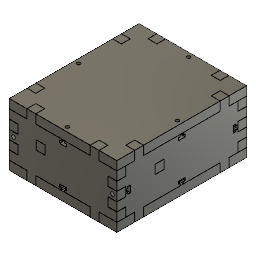
Basic-Case_1_ (Autodesk Fusion 360 design; units mm, degrees)
Autodesk Fusion 360 part; units mm, degrees
sketch "Sketch1" plane through (0, 0, 0) normal (0, 1, 0) x (1, 0, 0)
  line L0 (20, -25) -> (-20, -25) construction
  line L1 (-20, -25) -> (-20, 25) construction
  line L2 (-20, 25) -> (20, 25) construction
  line L3 (20, 25) -> (20, -25) construction
  line L4 (20, -25) -> (-20, 25) construction
  line L5 (-20, -25) -> (20, 25) construction
  line L6 (-20.2, -25.2) -> (-20.2, 25.2)
  line L7 (-20.2, 25.2) -> (20.2, 25.2)
  line L8 (20.2, 25.2) -> (20.2, -25.2)
  line L9 (20.2, -25.2) -> (-20.2, -25.2)
  line L10 (-24.2, -29.2) -> (-24.2, 29.2)
  line L11 (-24.2, 29.2) -> (24.2, 29.2)
  line L12 (24.2, 29.2) -> (24.2, -29.2)
  line L13 (24.2, -29.2) -> (-24.2, -29.2)
  line L14 (-101.376, 37.6811) -> (-97.376, 37.6811)
  circle A0 centre (-145.6614, -116.3344) radius 0.8
  line L15 (-102.0936, 18.9478) -> (-98.0936, 18.9478) construction
  line L16 (-115.2743, 43.6415) -> (-83.6806, 43.6415) construction
  line L17 (-83.6806, 43.6415) -> (-83.6806, 47.6415) construction
  line L18 (-83.6806, 47.6415) -> (-115.2743, 47.6415) construction
  line L19 (-115.2743, 47.6415) -> (-115.2743, 43.6415) construction
  line L20 (-141.8809, -116.5884) -> (-121.0391, -116.5884) construction
  line L21 (-121.0391, -116.5884) -> (-121.0391, -112.5884) construction
  line L22 (-121.0391, -112.5884) -> (-141.8809, -112.5884) construction
  line L23 (-141.8809, -112.5884) -> (-141.8809, -116.5884) construction
  line L24 (-113.6442, 20.144) -> (-90.9391, 20.144) construction
  line L25 (-90.9391, 20.144) -> (-90.9391, 24.144) construction
  line L26 (-90.9391, 24.144) -> (-113.6442, 24.144) construction
  line L27 (-113.6442, 24.144) -> (-113.6442, 20.144) construction
  line L28 (-117.1274, 62.4181) -> (-97.1274, 62.4181) construction
  line L29 (-106.7649, 64.5631) -> (-88.5969, 64.5631) construction
  line L30 (-88.5969, 64.5631) -> (-88.5969, 68.5631) construction
  line L31 (-88.5969, 68.5631) -> (-106.7649, 68.5631) construction
  line L32 (-106.7649, 68.5631) -> (-106.7649, 64.5631) construction
  line L33 (-131.4609, -76.5113) -> (-128.4609, -76.5113) construction
  line L34 (-133.0423, -91.4513) -> (-131.8423, -91.4513) construction
  line L35 (-127.3164, -91.6771) -> (-110.039, -91.6771) construction
  line L36 (-110.039, -91.6771) -> (-110.039, -87.6771) construction
  line L37 (-110.039, -87.6771) -> (-127.3164, -87.6771) construction
  line L38 (-127.3164, -87.6771) -> (-127.3164, -91.6771) construction
  line L39 (-126.3991, -76.4909) -> (-110.9245, -76.4909) construction
  line L40 (-110.9245, -76.4909) -> (-110.9245, -72.4909) construction
  line L41 (-110.9245, -72.4909) -> (-126.3991, -72.4909) construction
  line L42 (-126.3991, -72.4909) -> (-126.3991, -76.4909) construction
  line L43 (-135.3666, -105.8982) -> (-129.2666, -105.8982) construction
  line L44 (-125.3145, -106.1826) -> (-103.254, -106.1826) construction
  line L45 (-103.254, -106.1826) -> (-103.254, -102.1826) construction
  line L46 (-103.254, -102.1826) -> (-125.3145, -102.1826) construction
  line L47 (-125.3145, -102.1826) -> (-125.3145, -106.1826) construction
  dimension "d1" = 50
  dimension "d2" = 40
  dimension "d3" = 0.2
  dimension "d4" = 4.2
  dimension "d9" = 4
  dimension "d141" = 1.6
  dimension "d199" = 4
  dimension "d225" = 20
  dimension "d273" = 6.1
  dimension "d274" = 1.2
  dimension "d275" = 3
  constraint perpendicular L0 L1
  constraint parallel L0 L2
  constraint parallel L1 L3
  constraint horizontal L0
  constraint coincident L4 origin
  constraint coincident L5 origin
  constraint horizontal L14
  constraint horizontal L15
  constraint perpendicular L16 L17
  constraint parallel L16 L18
  constraint parallel L17 L19
  constraint perpendicular L20 L21
  constraint parallel L20 L22
  constraint parallel L21 L23
  constraint perpendicular L24 L25
  constraint parallel L24 L26
  constraint parallel L25 L27
  constraint horizontal L28
  constraint perpendicular L29 L30
  constraint parallel L29 L31
  constraint parallel L30 L32
  constraint horizontal L33
  constraint horizontal L34
  constraint perpendicular L35 L36
  constraint parallel L35 L37
  constraint parallel L36 L38
  constraint perpendicular L39 L40
  constraint parallel L39 L41
  constraint parallel L40 L42
  constraint horizontal L43
  constraint perpendicular L44 L45
  constraint parallel L44 L46
  constraint parallel L45 L47
  measures "d1" distance of L0.start L2.end
  measures "d2" distance of L0.start L0.end
  measures "d9" distance of L14.start L14.end
  measures "d141" diameter of A0
  measures "d199" distance of L15.start L15.end
  measures "d225" distance of L28.start L28.end
  measures "d273" distance of L43.start L43.end
  measures "d274" distance of L34.start L34.end
  measures "d275" distance of L33.start L33.end
extrude "Extrude1" add sketch "Sketch1" against normal blind 4 contours L6 L7 L8 L9 | L10 L11 L12 L13 makes body 1
extrude "Extrude3" add sketch "Sketch1" along normal blind 20 separate body contours L10 L11 L12 L13 makes body 2
sketch "Sketch2" plane through (0, 20, 0) normal (0, 1, 0) x (-1, 0, 0)
  line L0 (-20.2, -25.2) -> (-20.2, 25.2)
  line L1 (-20.2, 25.2) -> (20.2, 25.2)
  line L2 (20.2, 25.2) -> (20.2, -25.2)
  line L3 (20.2, -25.2) -> (-20.2, -25.2)
  line L4 (-24.2, 29.2) -> (-24.2, -29.2)
  line L5 (-24.2, -29.2) -> (24.2, -29.2)
  line L6 (24.2, -29.2) -> (24.2, 29.2)
  line L7 (24.2, 29.2) -> (-24.2, 29.2)
  line L8 (20.2, -25.2) -> (24.2, -29.2) construction
  line L9 (-20.2, -25.2) -> (-24.2, -29.2) construction
  line L10 (-20.2, 25.2) -> (-24.2, 29.2) construction
  line L11 (20.2, 25.2) -> (24.2, 29.2) construction
  circle A0 centre (22.2, 27.2) radius 0.75
  circle A1 centre (-22.2, 27.2) radius 0.75
  circle A2 centre (-22.2, -27.2) radius 0.75
  circle A3 centre (22.2, -27.2) radius 0.75
  dimension "d95" = 1.5
  dimension "d96" = 1.5
  dimension "d97" = 1.5
  dimension "d98" = 1.5
  constraint coincident L2.end L3.start
  constraint coincident L5.end L6.start
  constraint coincident L0.start L3.end
  constraint coincident L4.end L5.start
  constraint coincident L0.end L1.start
  constraint coincident L4.start L7.end
  constraint coincident L1.end L2.start
  constraint coincident L6.end L7.start
  constraint midpoint L11 A0.centre
  constraint midpoint L10 A1.centre
  constraint midpoint L9 A2.centre
  constraint midpoint L8 A3.centre
  measures "d95" diameter of A0
  measures "d96" diameter of A1
  measures "d97" diameter of A2
  measures "d98" diameter of A3
extrude "Extrude4" add sketch "Sketch2" along normal blind 4 separate body contours L0 L1 L2 L3 | L4 L5 L6 L7 | A0 | A1 | A2 | A3 makes body 3
sketch "Sketch7" plane through (0, 20, 0) normal (0, 1, 0) x (-1, 0, 0)
  line L0 (24.2, -29.2) -> (24.2, 29.2)
  line L1 (24.2, 29.2) -> (-24.2, 29.2)
  line L2 (-24.2, 29.2) -> (-24.2, -29.2)
  line L3 (-24.2, -29.2) -> (24.2, -29.2)
  line L4 (-20.2, -25.2) -> (-20.2, 25.2)
  line L5 (-20.2, 25.2) -> (20.2, 25.2)
  line L6 (20.2, 25.2) -> (20.2, -25.2)
  line L7 (20.2, -25.2) -> (-20.2, -25.2)
  line L8 (-12.2, -25.2) -> (-16.2, -25.2)
  line L9 (-16.2, -25.2) -> (-16.2, -29.2)
  line L10 (-16.2, -29.2) -> (-12.2, -29.2)
  line L11 (-12.2, -29.2) -> (-12.2, -25.2)
  line L12 (-24.2, -17.2) -> (-20.2, -17.2)
  line L13 (-20.2, -17.2) -> (-20.2, -21.2)
  line L14 (-20.2, -21.2) -> (-24.2, -21.2)
  line L15 (-24.2, -21.2) -> (-24.2, -17.2)
  line L16 (-24.2, 21.2) -> (-20.2, 21.2)
  line L17 (-24.2, 17.2) -> (-20.2, 17.2)
  line L18 (-16.2, 25.2) -> (-16.2, 29.2)
  line L19 (-12.2, 29.2) -> (-12.2, 25.2)
  line L20 (16.2, 29.2) -> (16.2, 25.2)
  line L21 (12.2, 25.2) -> (12.2, 29.2)
  line L22 (20.2, 21.2) -> (24.2, 21.2)
  line L23 (24.2, 17.2) -> (20.2, 17.2)
  line L24 (12.2, -25.2) -> (12.2, -29.2)
  line L25 (16.2, -25.2) -> (16.2, -29.2)
  line L26 (20.2, -21.2) -> (24.2, -21.2)
  line L27 (24.2, -17.2) -> (20.2, -17.2)
  line L28 (24.2, 0) -> (-24.2, 0) construction
  dimension "d74" = 4
  dimension "d75" = 4
  dimension "d76" = 4
  dimension "d77" = 4
  dimension "d78" = 4
  dimension "d79" = 4
  dimension "d80" = 4
  dimension "d81" = 4
  dimension "d82" = 4
  dimension "d83" = 4
  dimension "d84" = 4
  dimension "d85" = 4
  dimension "d86" = 4
  dimension "d87" = 4
  dimension "d88" = 4
  dimension "d198" = 4
  constraint horizontal L8
  constraint vertical L9
  constraint horizontal L10
  constraint vertical L11
  constraint coincident L3 L9.end
  constraint horizontal L12
  constraint vertical L13
  constraint horizontal L14
  constraint vertical L15
  constraint coincident L4 L13.end
  constraint coincident L2 L12.start
  constraint coincident L2 L16.start
  constraint coincident L4 L16.end
  constraint coincident L2 L17.start
  constraint coincident L4 L17.end
  constraint coincident L5 L18.start
  constraint coincident L1 L18.end
  constraint coincident L1 L19.start
  constraint coincident L5 L19.end
  constraint coincident L1 L20.start
  constraint coincident L5 L20.end
  constraint coincident L5 L21.start
  constraint coincident L1 L21.end
  constraint coincident L6 L22.start
  constraint coincident L0 L22.end
  constraint coincident L0 L23.start
  constraint coincident L6 L23.end
  constraint coincident L7 L24.start
  constraint coincident L7 L25.start
  constraint coincident L6 L26.start
  constraint coincident L0 L26.end
  constraint coincident L0 L27.start
  constraint coincident L6 L27.end
  constraint vertical L24
  constraint vertical L25
  constraint horizontal L26
  constraint horizontal L27
  constraint horizontal L22
  constraint horizontal L23
  constraint vertical L20
  constraint vertical L21
  constraint vertical L18
  constraint vertical L19
  constraint horizontal L16
  constraint horizontal L17
  constraint coincident L3 L24.end
  constraint coincident L3 L25.end
  constraint coincident L7 L8.start
  constraint midpoint L0 L28.start
  constraint midpoint L2 L28.end
  measures "d74" distance of L9 L11
  measures "d75" distance of L4.start L9
  measures "d76" distance of L4.start L14
  measures "d77" distance of L12 L14
  measures "d78" distance of L16 L17
  measures "d79" distance of L4.end L16
  measures "d80" distance of L18 L19
  measures "d81" distance of L4.end L18
  measures "d82" distance of L5.end L20
  measures "d83" distance of L20 L21
  measures "d84" distance of L5.end L22
  measures "d85" distance of L22 L23
  measures "d86" distance of L24 L25
  measures "d87" distance of L26 L27
  measures "d88" distance of L6.end L26
  measures "d198" distance of L6.end L25
extrude "Extrude37" add sketch "Sketch7" against normal blind 4 from surface at -20 contours L0 L6 L26 L27 | L3 L7 L24 L25 | L0 L6 L22 L23 | L3 L7 L8 L9 L10 L11 | L1 L5 L20 L21 | L2 L4 L12 L13 L14 L15 | L1 L5 L18 L19 | L2 L4 L16 L17 bodies 2
extrude "Extrude11" add sketch "Sketch7" along normal blind 4 contours L0 L6 L26 L27 | L3 L7 L24 L25 | L0 L6 L22 L23 | L3 L7 L8 L9 L10 L11 | L1 L5 L20 L21 | L2 L4 L12 L13 L14 L15 | L1 L5 L18 L19 | L2 L4 L16 L17 bodies 2
sketch "Sketch25" plane through (0, 20, 0) normal (0, 1, 0) x (-1, 0, 0)
  line L0 (24.2, 17.2) -> (20.2, 17.2)
  line L1 (20.2, 17.2) -> (20.2, -17.2)
  line L2 (20.2, -17.2) -> (24.2, -17.2)
  line L3 (24.2, -17.2) -> (24.2, 17.2)
  line L4 (24.2, -17.25) -> (20.2, -17.25)
  line L5 (24.2, -21.15) -> (20.2, -21.15)
  line L6 (16.15, -44.2) -> (16.15, -40.2)
  line L7 (12.25, -44.2) -> (12.25, -40.2)
  line L8 (-12.25, -44.2) -> (-12.25, -40.2)
  line L9 (-16.15, -44.2) -> (-16.15, -40.2)
  line L10 (-20.2, -21.15) -> (-24.2, -21.15)
  line L11 (-24.2, -17.25) -> (-20.2, -17.25)
  line L12 (-20.2, 17.25) -> (-24.2, 17.25)
  line L13 (-20.2, 21.15) -> (-24.2, 21.15)
  line L14 (-16.15, 40.2) -> (-16.15, 44.2)
  line L15 (-12.25, 40.2) -> (-12.25, 44.2)
  line L16 (12.25, 40.2) -> (12.25, 44.2)
  line L17 (16.15, 40.2) -> (16.15, 44.2)
  line L18 (24.2, 21.15) -> (20.2, 21.15)
  line L19 (24.2, 17.25) -> (20.2, 17.25)
  line L20 (24.2, -21.2) -> (20.2, -21.2)
  line L21 (16.2, -25.2) -> (16.2, -29.2)
  line L22 (12.2, -29.2) -> (12.2, -25.2)
  line L23 (-12.2, -25.2) -> (-12.2, -29.2)
  line L24 (-20.2, -21.2) -> (-24.2, -21.2)
  line L25 (-24.2, -17.2) -> (-20.2, -17.2)
  line L26 (-16.2, -29.2) -> (-16.2, -25.2)
  line L27 (-20.2, 17.2) -> (-24.2, 17.2)
  line L28 (-24.2, 21.2) -> (-20.2, 21.2)
  line L29 (-16.2, 25.2) -> (-16.2, 29.2)
  line L30 (-12.2, 29.2) -> (-12.2, 25.2)
  line L31 (12.2, 25.2) -> (12.2, 29.2)
  line L32 (16.2, 29.2) -> (16.2, 25.2)
  line L33 (20.2, 21.2) -> (24.2, 21.2)
  line L34 (-16.2, -29.2) -> (-24.2, -29.2)
  line L35 (12.2, -29.2) -> (-12.2, -29.2)
  line L36 (-16.2, -25.2) -> (-20.2, -25.2)
  line L37 (12.2, -25.2) -> (-12.2, -25.2)
  line L38 (-20.2, 21.2) -> (-20.2, 25.2)
  line L39 (-20.2, -17.2) -> (-20.2, 17.2)
  line L40 (-24.2, 21.2) -> (-24.2, 29.2)
  line L41 (-24.2, -17.2) -> (-24.2, 17.2)
  line L42 (16.2, 25.2) -> (20.2, 25.2)
  line L43 (-12.2, 25.2) -> (12.2, 25.2)
  line L44 (16.2, 29.2) -> (24.2, 29.2)
  line L45 (-12.2, 29.2) -> (12.2, 29.2)
  line L46 (24.2, -21.2) -> (24.2, -29.2)
  line L47 (24.2, 17.2) -> (24.2, -17.2)
  line L48 (20.2, -21.2) -> (20.2, -25.2)
  line L49 (20.2, 17.2) -> (20.2, -17.2)
  line L50 (24.2, -29.2) -> (16.2, -29.2)
  line L51 (20.2, -25.2) -> (16.2, -25.2)
  line L52 (-20.2, -25.2) -> (-20.2, -21.2)
  line L53 (-24.2, -29.2) -> (-24.2, -21.2)
  line L54 (-20.2, 25.2) -> (-16.2, 25.2)
  line L55 (-24.2, 29.2) -> (-16.2, 29.2)
  line L56 (24.2, 29.2) -> (24.2, 21.2)
  line L57 (20.2, 25.2) -> (20.2, 21.2)
  dimension "d238" = 0.05
  dimension "d239" = 0.05
  dimension "d240" = 0.05
  dimension "d241" = 0.05
  dimension "d242" = 0.05
  dimension "d243" = 0.05
  dimension "d244" = 0.05
  dimension "d245" = 0.05
  dimension "d246" = 0.05
  dimension "d247" = 0.05
  dimension "d248" = 0.05
  dimension "d249" = 0.05
  dimension "d250" = 0.05
  dimension "d251" = 0.05
  dimension "d252" = 0.05
  dimension "d253" = 0.05
  constraint coincident L3 L4.start
  constraint coincident L1 L4.end
  constraint perpendicular L1 L4
  constraint perpendicular L1 L5
  constraint perpendicular L9 L10
  constraint perpendicular L13 L14
  constraint perpendicular L17 L18
  measures "d238" distance of L2 L4
  measures "d239" distance of L5 L20
  measures "d240" distance of L6 L21
  measures "d241" distance of L7 L22
  measures "d242" distance of L8 L23
  measures "d243" distance of L10 L24
  measures "d244" distance of L11 L25
  measures "d245" distance of L9 L26
  measures "d246" distance of L12 L27
  measures "d247" distance of L13 L28
  measures "d248" distance of L14 L29
  measures "d249" distance of L15 L30
  measures "d250" distance of L16 L31
  measures "d251" distance of L17 L32
  measures "d252" distance of L18 L33
  measures "d253" distance of L0 L19
extrude "Extrude36" cut sketch "Sketch7" along normal through all and the other way through all contours L0 L6 L26 L27 | L3 L7 L24 L25 | L0 L6 L22 L23 | L3 L7 L8 L9 L10 L11 | L1 L5 L20 L21 | L2 L4 L12 L13 L14 L15 | L1 L5 L18 L19 | L2 L4 L16 L17 bodies 1 3
split "Split7" by plane through (-20.2, 0, -25.2) normal (0, 0, 1) bodies 2 makes body 4 at (-24.2, 13.3333, 5.7333)
split "Split8" by plane through (20.2, 0, 25.2) normal (0, 0, -1) bodies 4 makes body 5 at (20.2, 13.3333, 5.7333) makes body 6 at (-24.2, 13.3333, -5.7333)
sketch "Sketch24" plane through (0, 0, 25.2) normal (0, 0, 1) x (1, 0, 0)
  line L0 (24.2, 0) -> (24.2, 20)
  line L1 (20.2, 16) -> (24.2, 16)
  line L2 (24.2, 12) -> (20.2, 12)
  line L3 (20.2, 8) -> (24.2, 8)
  line L4 (24.2, 4) -> (20.2, 4)
  line L5 (-24.2, 16) -> (-20.2, 16)
  line L6 (-20.2, 16) -> (-20.2, 12)
  line L7 (-20.2, 12) -> (-24.2, 12)
  line L8 (-24.2, 12) -> (-24.2, 16)
  line L9 (-24.2, 8) -> (-20.2, 8)
  line L10 (-20.2, 8) -> (-20.2, 4)
  line L11 (-20.2, 4) -> (-24.2, 4)
  line L12 (-24.2, 4) -> (-24.2, 8)
  line L13 (-24.2, 20) -> (-24.2, 0)
  line L14 (-24.2, 0) -> (-24.2, 20)
  line L15 (24.2, 12) -> (24.2, 16)
  line L16 (20.2, 16) -> (20.2, 12)
  line L17 (20.2, 8) -> (20.2, 4)
  line L18 (24.2, 0) -> (20.2, 0)
  line L19 (20.2, 20) -> (24.2, 20)
  dimension "d231" = 4
  dimension "d296" = 4
  dimension "d298" = 4
  dimension "d299" = 4
  dimension "d300" = 4
  dimension "d301" = 4
  dimension "d303" = 4
  dimension "d304" = 4
  constraint perpendicular L0 L3
  constraint coincident L0 L4.start
  constraint perpendicular L0 L4
  constraint horizontal L5
  constraint vertical L6
  constraint horizontal L7
  constraint vertical L8
  constraint horizontal L9
  constraint vertical L10
  constraint horizontal L11
  constraint vertical L12
  constraint collinear L1 L5
  constraint collinear L2 L7
  constraint collinear L3 L9
  constraint collinear L4 L11
  constraint collinear L8 L14
  constraint collinear L12 L14
  constraint collinear L0 L15
  constraint vertical L16
  constraint perpendicular L4 L17
  constraint coincident L0 L3.end
  measures "d231" distance of L1 L2
  measures "d296" distance of L3 L4
  measures "d298" distance of L1.start L1.end
  measures "d299" distance of L5.start L5.end
  measures "d300" distance of L4.start L4.end
  measures "d301" distance of L10.end L11.end
  measures "d303" distance of L4 L18
  measures "d304" distance of L1 L19
extrude "Extrude35" add sketch "Sketch24" along normal blind 4 bodies 5 6
mirror "Mirror5" about plane through (0, 0, 0) normal (0, 0, 1) of "Extrude35"
sketch "Sketch26" plane through (0, 0, 29.2) normal (0, 0, 1) x (1, 0, 0)
  line L0 (16.2, 0) -> (24.2, 0)
  line L1 (24.2, 0) -> (24.2, 20)
  line L2 (24.2, 20) -> (16.2, 20)
  line L3 (16.2, 20) -> (16.2, 24)
  line L4 (16.2, 24) -> (12.2, 24)
  line L5 (12.2, 24) -> (12.2, 20)
  line L6 (12.2, 20) -> (-12.2, 20)
  line L7 (-12.2, 20) -> (-12.2, 24)
  line L8 (-12.2, 24) -> (-16.2, 24)
  line L9 (-16.2, 24) -> (-16.2, 20)
  line L10 (-16.2, 20) -> (-24.2, 20)
  line L11 (-24.2, 20) -> (-24.2, 0)
  line L12 (-24.2, 0) -> (-16.2, 0)
  line L13 (-16.2, 0) -> (-16.2, -4)
  line L14 (-16.2, -4) -> (-12.2, -4)
  line L15 (-12.2, -4) -> (-12.2, 0)
  line L16 (-12.2, 0) -> (12.2, 0)
  line L17 (12.2, 0) -> (12.2, -4)
  line L18 (12.2, -4) -> (16.2, -4)
  line L19 (16.2, -4) -> (16.2, 0)
  line L20 (24.2, 16) -> (20.2, 16)
  line L21 (20.2, 12) -> (24.2, 12)
  line L22 (24.2, 8) -> (20.2, 8)
  line L23 (20.2, 4) -> (24.2, 4)
  line L24 (20.2, 16) -> (20.2, 12)
  line L25 (24.2, 16) -> (24.2, 12)
  line L26 (20.2, 8) -> (20.2, 4)
  line L27 (24.2, 8) -> (24.2, 4)
  line L28 (0, 0) -> (0, 17.3117) construction
  line L29 (20.2, 15.95) -> (24.2, 15.95)
  line L30 (24.2, 12.05) -> (20.2, 12.05)
  line L31 (20.2, 7.95) -> (24.2, 7.95)
  line L32 (24.2, 4.05) -> (20.2, 4.05)
  line L33 (-20.2, 7.95) -> (-24.2, 7.95)
  line L34 (-20.2, 8) -> (-20.2, 4)
  line L35 (-24.2, 8) -> (-24.2, 4)
  line L36 (-24.2, 4.05) -> (-20.2, 4.05)
  line L37 (-20.2, 15.95) -> (-24.2, 15.95)
  line L38 (-20.2, 16) -> (-20.2, 12)
  line L39 (-24.2, 12.05) -> (-20.2, 12.05)
  line L40 (-24.2, 16) -> (-24.2, 12)
  dimension "d260" = 0.05
  dimension "d261" = 0.05
  dimension "d262" = 0.05
  dimension "d263" = 0.05
  constraint coincident L20.end L24.start
  constraint coincident L21.start L24.end
  constraint coincident L20.start L25.start
  constraint coincident L21.end L25.end
  constraint coincident L22.end L26.start
  constraint coincident L23.start L26.end
  constraint coincident L22.start L27.start
  constraint coincident L23.end L27.end
  constraint coincident L28.start origin
  constraint vertical L28
  constraint coincident L24 L29.start
  constraint coincident L25 L29.end
  constraint coincident L25 L30.start
  constraint coincident L24 L30.end
  constraint perpendicular L24 L30
  constraint perpendicular L24 L29
  constraint coincident L26 L31.start
  constraint coincident L27 L31.end
  constraint coincident L27 L32.start
  constraint coincident L26 L32.end
  constraint perpendicular L26 L32
  constraint perpendicular L26 L31
  constraint symmetric L20.end L28 L38.start
  constraint symmetric L21.start L28 L38.end
  constraint symmetric L20.start L28 L40.start
  constraint symmetric L21.end L28 L40.end
  constraint symmetric L22.end L28 L34.start
  constraint symmetric L23.start L28 L34.end
  constraint symmetric L22.start L28 L35.start
  constraint symmetric L23.end L28 L35.end
  constraint symmetric L28 L29.start L37.start
  constraint symmetric L28 L29.end L37.end
  constraint symmetric L28 L30.start L39.start
  constraint symmetric L28 L30.end L39.end
  constraint symmetric L28 L31.start L33.start
  constraint symmetric L28 L31.end L33.end
  constraint symmetric L28 L32.start L36.start
  constraint symmetric L28 L32.end L36.end
  measures "d260" distance of L20 L29
  measures "d261" distance of L21 L30
  measures "d262" distance of L22 L31
  measures "d263" distance of L23 L32
extrude "Extrude38" cut sketch "Sketch26" against normal through all contours L1 L26 L27 L31 L32 | L1 L24 L25 L29 L30 | L11 L33 L34 L35 L36 | L11 L37 L38 L39 L40 bodies 2 4
sketch "Sketch10" plane through (0, -4, 0) normal (0, -1, 0) x (1, 0, 0)
  line L0 (-12.2, -29.2) -> (12.2, -29.2)
  line L1 (24.2, -29.2) -> (24.2, -21.2)
  line L2 (24.2, 29.2) -> (16.2, 29.2)
  line L3 (-24.2, 29.2) -> (-24.2, 21.2)
  line L4 (-20.2, 25.2) -> (-20.2, -25.2) construction
  line L5 (-20.2, 25.2) -> (20.2, 25.2) construction
  line L6 (20.2, 25.2) -> (20.2, -25.2) construction
  line L7 (20.2, -25.2) -> (-20.2, -25.2) construction
  circle A0 centre (0, 27.2) radius 0.75
  circle A1 centre (0, -27.2) radius 0.75
  line L8 (20.2, 0) -> (24.2, 0) construction
  circle A2 centre (22.2, 0) radius 0.75
  line L9 (-24.2, 0) -> (-20.2, 0) construction
  circle A3 centre (-22.2, 0) radius 0.75
  line L10 (-12.2, -25.2) -> (-12.2, -29.2)
  line L11 (12.2, -29.2) -> (12.2, -25.2)
  line L12 (12.2, -25.2) -> (16.2, -25.2)
  line L13 (16.2, -25.2) -> (16.2, -29.2)
  line L14 (16.2, -29.2) -> (24.2, -29.2)
  line L15 (24.2, -21.2) -> (20.2, -21.2)
  line L16 (20.2, -21.2) -> (20.2, -17.2)
  line L17 (20.2, -17.2) -> (24.2, -17.2)
  line L18 (24.2, -17.2) -> (24.2, 17.2)
  line L19 (24.2, 17.2) -> (20.2, 17.2)
  line L20 (20.2, 17.2) -> (20.2, 21.2)
  line L21 (20.2, 21.2) -> (24.2, 21.2)
  line L22 (24.2, 21.2) -> (24.2, 29.2)
  line L23 (16.2, 29.2) -> (16.2, 25.2)
  line L24 (16.2, 25.2) -> (12.2, 25.2)
  line L25 (12.2, 25.2) -> (12.2, 29.2)
  line L26 (12.2, 29.2) -> (-12.2, 29.2)
  line L27 (-12.2, 29.2) -> (-12.2, 25.2)
  line L28 (-12.2, 25.2) -> (-16.2, 25.2)
  line L29 (-16.2, 25.2) -> (-16.2, 29.2)
  line L30 (-16.2, 29.2) -> (-24.2, 29.2)
  line L31 (-24.2, 21.2) -> (-20.2, 21.2)
  line L32 (-20.2, 21.2) -> (-20.2, 17.2)
  line L33 (-20.2, 17.2) -> (-24.2, 17.2)
  line L34 (-24.2, 17.2) -> (-24.2, -17.2)
  line L35 (-24.2, -17.2) -> (-20.2, -17.2)
  line L36 (-20.2, -17.2) -> (-20.2, -21.2)
  line L37 (-20.2, -21.2) -> (-24.2, -21.2)
  line L38 (-24.2, -21.2) -> (-24.2, -29.2)
  line L39 (-24.2, -29.2) -> (-16.2, -29.2)
  line L40 (-16.2, -29.2) -> (-16.2, -25.2)
  line L41 (-16.2, -25.2) -> (-12.2, -25.2)
  line L42 (0, 25.2) -> (0, 29.2) construction
  line L43 (0, -29.2) -> (0, -25.2) construction
  point P0 (20.2, 25.2)
  point P1 (20.2, -25.2)
  point P2 (-20.2, -25.2)
  point P3 (-20.2, 25.2)
  point P4 (20.2, -21.2)
  point P5 (20.2, 21.2)
  point P6 (20.2, -17.2)
  point P7 (20.2, 17.2)
  point P8 (-20.2, -17.2)
  point P9 (-20.2, 21.2)
  point P10 (-20.2, 17.2)
  point P11 (-20.2, -21.2)
  dimension "d105" = 1.5
  dimension "d107" = 1.5
  dimension "d124" = 1.5
  dimension "d127" = 1.5
  constraint perpendicular L4 L5
  constraint perpendicular L6 L7
  constraint perpendicular L4 L7
  constraint coincident L6 L8.start
  constraint horizontal L8
  constraint coincident L4 L9.end
  constraint horizontal L9
  constraint midpoint L4 L9.end
  constraint midpoint L9 A3.centre
  constraint midpoint L6 L8.start
  constraint midpoint L8 A2.centre
  constraint midpoint L5 L42.start
  constraint midpoint L26 L42.end
  constraint perpendicular L26 L42
  constraint midpoint A0.centre L42
  constraint midpoint L0 L43.start
  constraint midpoint L7 L43.end
  constraint perpendicular L7 L43
  constraint midpoint A1.centre L43
  constraint midpoint L9.start L34
  constraint midpoint L8.end L18
  constraint coincident P3 L4.start
  measures "d105" diameter of A0
  measures "d107" diameter of A1
  measures "d124" diameter of A2
  measures "d127" diameter of A3
extrude "Extrude33" cut sketch "Sketch10" against normal blind 4 contours A0 | A1 | A2 | A3 bodies 1
sketch "Sketch23" plane through (0, 24, 0) normal (0, 1, 0) x (-1, 0, 0)
  line L0 (-24.2, 17.2) -> (-24.2, -17.2)
  line L1 (16.2, -29.2) -> (24.2, -29.2)
  line L2 (24.2, -29.2) -> (24.2, -21.2)
  line L3 (24.2, 29.2) -> (16.2, 29.2)
  line L4 (-24.2, 29.2) -> (-24.2, 21.2)
  circle A0 centre (0, 27.2) radius 0.75
  circle A1 centre (22.2, 0) radius 0.75
  circle A2 centre (-22.2, 0) radius 0.75
  line L5 (16.2, -25.2) -> (16.2, -29.2)
  line L6 (24.2, -21.2) -> (20.2, -21.2)
  line L7 (20.2, -21.2) -> (20.2, -17.2)
  line L8 (20.2, -17.2) -> (24.2, -17.2)
  line L9 (24.2, -17.2) -> (24.2, 17.2)
  line L10 (24.2, 17.2) -> (20.2, 17.2)
  line L11 (20.2, 17.2) -> (20.2, 21.2)
  line L12 (20.2, 21.2) -> (24.2, 21.2)
  line L13 (24.2, 21.2) -> (24.2, 29.2)
  line L14 (16.2, 29.2) -> (16.2, 25.2)
  line L15 (16.2, 25.2) -> (12.2, 25.2)
  line L16 (12.2, 25.2) -> (12.2, 29.2)
  line L17 (12.2, 29.2) -> (-12.2, 29.2)
  line L18 (-12.2, 29.2) -> (-12.2, 25.2)
  line L19 (-12.2, 25.2) -> (-16.2, 25.2)
  line L20 (-16.2, 25.2) -> (-16.2, 29.2)
  line L21 (-16.2, 29.2) -> (-24.2, 29.2)
  line L22 (-24.2, 21.2) -> (-20.2, 21.2)
  line L23 (-20.2, 21.2) -> (-20.2, 17.2)
  line L24 (-20.2, 17.2) -> (-24.2, 17.2)
  line L25 (-24.2, -17.2) -> (-20.2, -17.2)
  line L26 (-20.2, -17.2) -> (-20.2, -21.2)
  line L27 (-20.2, -21.2) -> (-24.2, -21.2)
  line L28 (-24.2, -21.2) -> (-24.2, -29.2)
  line L29 (-24.2, -29.2) -> (-16.2, -29.2)
  line L30 (-16.2, -29.2) -> (-16.2, -25.2)
  line L31 (-16.2, -25.2) -> (-12.2, -25.2)
  line L32 (-12.2, -25.2) -> (-12.2, -29.2)
  line L33 (-12.2, -29.2) -> (12.2, -29.2)
  line L34 (12.2, -29.2) -> (12.2, -25.2)
  line L35 (12.2, -25.2) -> (16.2, -25.2)
  circle A3 centre (0, -27.2) radius 0.75
extrude "Extrude34" cut sketch "Sketch23" against normal blind 4 contours A0 | A1 | A2 | A3 bodies 3
sketch "Sketch27" plane through (0, 0, 29.2) normal (0, 0, 1) x (1, 0, 0)
  line L0 (20.2, 7.95) -> (24.2, 7.95)
  line L1 (24.2, 7.95) -> (24.2, 12.05)
  line L2 (24.2, 12.05) -> (20.2, 12.05)
  line L3 (20.2, 12.05) -> (20.2, 15.95)
  line L4 (20.2, 15.95) -> (24.2, 15.95)
  line L5 (24.2, 15.95) -> (24.2, 20)
  line L6 (24.2, 20) -> (16.2, 20)
  line L7 (16.2, 20) -> (16.2, 24)
  line L8 (16.2, 24) -> (12.2, 24)
  line L9 (12.2, 24) -> (12.2, 20)
  line L10 (12.2, 20) -> (-12.2, 20)
  line L11 (-12.2, 20) -> (-12.2, 24)
  line L12 (-12.2, 24) -> (-16.2, 24)
  line L13 (-16.2, 24) -> (-16.2, 20)
  line L14 (-16.2, 20) -> (-24.2, 20)
  line L15 (-24.2, 20) -> (-24.2, 15.95)
  line L16 (-24.2, 15.95) -> (-20.2, 15.95)
  line L17 (-20.2, 15.95) -> (-20.2, 12.05)
  line L18 (-20.2, 12.05) -> (-24.2, 12.05)
  line L19 (-24.2, 12.05) -> (-24.2, 7.95)
  line L20 (-24.2, 7.95) -> (-20.2, 7.95)
  line L21 (-20.2, 7.95) -> (-20.2, 4.05)
  line L22 (-20.2, 4.05) -> (-24.2, 4.05)
  line L23 (-24.2, 4.05) -> (-24.2, 0)
  line L24 (-24.2, 0) -> (-16.2, 0)
  line L25 (-16.2, 0) -> (-16.2, -4)
  line L26 (-16.2, -4) -> (-12.2, -4)
  line L27 (-12.2, -4) -> (-12.2, 0)
  line L28 (-12.2, 0) -> (12.2, 0)
  line L29 (12.2, 0) -> (12.2, -4)
  line L30 (12.2, -4) -> (16.2, -4)
  line L31 (16.2, -4) -> (16.2, 0)
  line L32 (16.2, 0) -> (24.2, 0)
  line L33 (24.2, 0) -> (24.2, 4.05)
  line L34 (24.2, 4.05) -> (20.2, 4.05)
  line L35 (20.2, 4.05) -> (20.2, 7.95)
  line L36 (-24.2, 12.05) -> (-20.2, 7.95) construction
  circle A0 centre (-22.2, 10) radius 0.8
  line L37 (0, 0) -> (0, 16.234) construction
  circle A1 centre (22.2, 10) radius 0.8
  dimension "d266" = 1.6
  constraint coincident L18.end L19.start
  constraint coincident L20.end L21.start
  constraint midpoint L36 A0.centre
  constraint coincident L37.start origin
  constraint vertical L37
  constraint symmetric A0 L37 A1
  measures "d266" diameter of A0
extrude "Extrude39" cut sketch "Sketch27" against normal blind 4 contours A0 | A1 bodies 4
sketch "Sketch28" plane through (0, 0, -29.2) normal (0, 0, -1) x (-1, 0, 0)
  line L0 (-24.2, 7.95) -> (-20.2, 7.95)
  line L1 (-20.2, 7.95) -> (-20.2, 4.05)
  line L2 (-20.2, 4.05) -> (-24.2, 4.05)
  line L3 (-24.2, 4.05) -> (-24.2, 0)
  line L4 (-24.2, 0) -> (-16.2, 0)
  line L5 (-16.2, 0) -> (-16.2, -4)
  line L6 (-16.2, -4) -> (-12.2, -4)
  line L7 (-12.2, -4) -> (-12.2, 0)
  line L8 (-12.2, 0) -> (12.2, 0)
  line L9 (12.2, 0) -> (12.2, -4)
  line L10 (12.2, -4) -> (16.2, -4)
  line L11 (16.2, -4) -> (16.2, 0)
  line L12 (16.2, 0) -> (24.2, 0)
  line L13 (24.2, 0) -> (24.2, 4.05)
  line L14 (24.2, 4.05) -> (20.2, 4.05)
  line L15 (20.2, 4.05) -> (20.2, 7.95)
  line L16 (20.2, 7.95) -> (24.2, 7.95)
  line L17 (24.2, 7.95) -> (24.2, 12.05)
  line L18 (24.2, 12.05) -> (20.2, 12.05)
  line L19 (20.2, 12.05) -> (20.2, 15.95)
  line L20 (20.2, 15.95) -> (24.2, 15.95)
  line L21 (24.2, 15.95) -> (24.2, 20)
  line L22 (24.2, 20) -> (16.2, 20)
  line L23 (16.2, 20) -> (16.2, 24)
  line L24 (16.2, 24) -> (12.2, 24)
  line L25 (12.2, 24) -> (12.2, 20)
  line L26 (12.2, 20) -> (-12.2, 20)
  line L27 (-12.2, 20) -> (-12.2, 24)
  line L28 (-12.2, 24) -> (-16.2, 24)
  line L29 (-16.2, 24) -> (-16.2, 20)
  line L30 (-16.2, 20) -> (-24.2, 20)
  line L31 (-24.2, 20) -> (-24.2, 15.95)
  line L32 (-24.2, 15.95) -> (-20.2, 15.95)
  line L33 (-20.2, 15.95) -> (-20.2, 12.05)
  line L34 (-20.2, 12.05) -> (-24.2, 12.05)
  line L35 (-24.2, 12.05) -> (-24.2, 7.95)
  circle A0 centre (22.2, 10) radius 0.8
  circle A1 centre (-22.2, 10) radius 0.8
extrude "Extrude40" cut sketch "Sketch28" against normal blind 4 contours A0 | A1 bodies 2
sketch "Sketch29" plane through (-24.2, 0, 0) normal (-1, 0, 0) x (0, 0, 1)
  line L0 (25.2, 0) -> (25.2, 4)
  line L1 (25.2, 4) -> (29.2, 4)
  line L2 (29.2, 4) -> (29.2, 8)
  line L3 (29.2, 8) -> (25.2, 8)
  line L4 (25.2, 8) -> (25.2, 12)
  line L5 (25.2, 12) -> (29.2, 12)
  line L6 (29.2, 12) -> (29.2, 16)
  line L7 (29.2, 16) -> (25.2, 16)
  line L8 (25.2, 16) -> (25.2, 20)
  line L9 (25.2, 20) -> (21.2, 20)
  line L10 (21.2, 20) -> (21.2, 24)
  line L11 (21.2, 24) -> (17.2, 24)
  line L12 (17.2, 24) -> (17.2, 20)
  line L13 (17.2, 20) -> (-17.2, 20)
  line L14 (-17.2, 20) -> (-17.2, 24)
  line L15 (-17.2, 24) -> (-21.2, 24)
  line L16 (-21.2, 24) -> (-21.2, 20)
  line L17 (-21.2, 20) -> (-25.2, 20)
  line L18 (-25.2, 20) -> (-25.2, 16)
  line L19 (-25.2, 16) -> (-29.2, 16)
  line L20 (-29.2, 16) -> (-29.2, 12)
  line L21 (-29.2, 12) -> (-25.2, 12)
  line L22 (-25.2, 12) -> (-25.2, 8)
  line L23 (-25.2, 8) -> (-29.2, 8)
  line L24 (-29.2, 8) -> (-29.2, 4)
  line L25 (-29.2, 4) -> (-25.2, 4)
  line L26 (-25.2, 4) -> (-25.2, 0)
  line L27 (-25.2, 0) -> (-21.2, 0)
  line L28 (-21.2, 0) -> (-21.2, -4)
  line L29 (-21.2, -4) -> (-17.2, -4)
  line L30 (-17.2, -4) -> (-17.2, 0)
  line L31 (-17.2, 0) -> (17.2, 0)
  line L32 (17.2, 0) -> (17.2, -4)
  line L33 (17.2, -4) -> (21.2, -4)
  line L34 (21.2, -4) -> (21.2, 0)
  line L35 (21.2, 0) -> (25.2, 0)
  line L36 (-0.75, 24) -> (0.75, 24)
  line L37 (0.75, -4) -> (-0.75, -4)
  line L38 (29.2, 10.8) -> (29.2, 9.2)
  line L39 (-29.2, 9.2) -> (-29.2, 10.8)
  line L40 (-25.2, 10.8) -> (-24.3, 10.8)
  line L41 (-24.3, 10.8) -> (-24.3, 11.5)
  line L42 (-24.3, 11.5) -> (-23.1, 11.5)
  line L43 (-23.1, 11.5) -> (-23.1, 8.5)
  line L44 (-23.1, 8.5) -> (-24.3, 8.5)
  line L45 (-24.3, 8.5) -> (-24.3, 9.2)
  line L46 (-24.3, 9.2) -> (-25.2, 9.2)
  line L47 (0.75, 20) -> (0.75, 19.1)
  line L48 (0.75, 19.1) -> (1.5, 19.1)
  line L49 (1.5, 19.1) -> (1.5, 17.9)
  line L50 (1.5, 17.9) -> (-1.5, 17.9)
  line L51 (-1.5, 17.9) -> (-1.5, 19.1)
  line L52 (-1.5, 19.1) -> (-0.75, 19.1)
  line L53 (-0.75, 19.1) -> (-0.75, 20)
  line L54 (-17.2, 24) -> (17.2, 24)
  line L55 (23.1, 11.5) -> (23.1, 8.5)
  line L56 (24.3, 11.5) -> (23.1, 11.5)
  line L57 (24.3, 10.8) -> (24.3, 11.5)
  line L58 (23.1, 8.5) -> (24.3, 8.5)
  line L59 (24.3, 8.5) -> (24.3, 9.2)
  line L60 (1.5, 0.9) -> (1.5, 2.1)
  line L61 (1.5, 2.1) -> (-1.5, 2.1)
  line L62 (-1.5, 2.1) -> (-1.5, 0.9)
  line L63 (-0.75, 0.9) -> (-0.75, 0)
  line L64 (-1.5, 0.9) -> (-0.75, 0.9)
  line L65 (0.75, 0) -> (0.75, 0.9)
  line L66 (0.75, 0.9) -> (1.5, 0.9)
  line L67 (24.3, 9.2) -> (25.2, 9.2)
  line L68 (24.3, 10.8) -> (25.2, 10.8)
  point P0 (25.2, 22.5)
  dimension "d272" = 3
  dimension "d276" = 6.1
  dimension "d277" = 1.2
  dimension "d278" = 3
  dimension "d279" = 1.2
  dimension "d280" = 6.1
  dimension "d281" = 6.1
  dimension "d282" = 1.2
  dimension "d283" = 3
  dimension "d284" = 3
  dimension "d285" = 1.2
  dimension "d286" = 6.1
  constraint coincident L22 L40.start
  constraint perpendicular L22 L40
  constraint perpendicular L40 L41
  constraint perpendicular L41 L42
  constraint perpendicular L42 L43
  constraint perpendicular L41 L44
  constraint perpendicular L44 L45
  constraint coincident L22 L46.end
  constraint perpendicular L22 L46
  constraint coincident L39.start L46
  constraint coincident L39.end L40
  constraint equal L41 L45
  constraint collinear L41 L45
  constraint coincident L13 L47.start
  constraint perpendicular L13 L47
  constraint perpendicular L47 L48
  constraint perpendicular L48 L49
  constraint perpendicular L47 L50
  constraint perpendicular L50 L51
  constraint perpendicular L51 L52
  constraint coincident L13 L53.end
  constraint perpendicular L13 L53
  constraint coincident L36.start L53
  constraint coincident L36.end L47
  constraint equal L48 L52
  constraint collinear L48 L52
  constraint collinear L64 L66
  constraint equal L64 L66
  constraint equal L57 L59
  constraint collinear L57 L59
  constraint perpendicular L60 L61
  constraint perpendicular L61 L62
  constraint perpendicular L62 L64
  constraint perpendicular L63 L64
  constraint perpendicular L65 L66
  constraint perpendicular L31 L65
  constraint perpendicular L55 L56
  constraint perpendicular L56 L57
  constraint perpendicular L55 L58
  constraint coincident L37.end L63
  constraint coincident L37.start L65
  constraint coincident L4 L67.end
  constraint perpendicular L4 L67
  constraint coincident L4 L68.end
  constraint perpendicular L4 L68
  constraint coincident L38.start L68
  constraint coincident L38.end L67
  measures "d272" distance of L42.end L43.end
  measures "d276" distance of L20 L43
  measures "d277" distance of L43.end L44.end
  measures "d278" distance of L49.end L50.end
  measures "d279" distance of L50.end L51.end
  measures "d280" distance of L50 L54
  measures "d281" distance of L38 L55
  measures "d282" distance of L55.start L56.start
  measures "d283" distance of L55.start L55.end
  measures "d284" distance of L60.end L61.end
  measures "d285" distance of L60.end L60.start
  measures "d286" distance of L37 L61
extrude "Extrude41" cut sketch "Sketch29" against normal through all contours L4 L55 L56 L57 L58 L59 L67 L68 | L31 L60 L61 L62 L63 L64 L65 L66 | L13 L47 L48 L49 L50 L51 L52 L53 | L22 L40 L41 L42 L43 L44 L45 L46 bodies 6 5
sketch "Sketch31" plane through (0, 0, 29.2) normal (0, 0, 1) x (1, 0, 0)
  circle A0 centre (-22.2, 10) radius 0.8
  circle A1 centre (22.2, 10) radius 0.8
  line L0 (20.2, 7.95) -> (24.2, 7.95)
  line L1 (24.2, 7.95) -> (24.2, 12.05)
  line L2 (24.2, 12.05) -> (20.2, 12.05)
  line L3 (20.2, 12.05) -> (20.2, 15.95)
  line L4 (20.2, 15.95) -> (24.2, 15.95)
  line L5 (24.2, 15.95) -> (24.2, 20)
  line L6 (24.2, 20) -> (16.2, 20)
  line L7 (16.2, 20) -> (16.2, 24)
  line L8 (16.2, 24) -> (12.2, 24)
  line L9 (12.2, 24) -> (12.2, 20)
  line L10 (12.2, 20) -> (-12.2, 20)
  line L11 (-12.2, 20) -> (-12.2, 24)
  line L12 (-12.2, 24) -> (-16.2, 24)
  line L13 (-16.2, 24) -> (-16.2, 20)
  line L14 (-16.2, 20) -> (-24.2, 20)
  line L15 (-24.2, 20) -> (-24.2, 15.95)
  line L16 (-24.2, 15.95) -> (-20.2, 15.95)
  line L17 (-20.2, 15.95) -> (-20.2, 12.05)
  line L18 (-20.2, 12.05) -> (-24.2, 12.05)
  line L19 (-24.2, 12.05) -> (-24.2, 7.95)
  line L20 (-24.2, 7.95) -> (-20.2, 7.95)
  line L21 (-20.2, 7.95) -> (-20.2, 4.05)
  line L22 (-20.2, 4.05) -> (-24.2, 4.05)
  line L23 (-24.2, 4.05) -> (-24.2, 0)
  line L24 (-24.2, 0) -> (-16.2, 0)
  line L25 (-16.2, 0) -> (-16.2, -4)
  line L26 (-16.2, -4) -> (-12.2, -4)
  line L27 (-12.2, -4) -> (-12.2, 0)
  line L28 (-12.2, 0) -> (12.2, 0)
  line L29 (12.2, 0) -> (12.2, -4)
  line L30 (12.2, -4) -> (16.2, -4)
  line L31 (16.2, -4) -> (16.2, 0)
  line L32 (16.2, 0) -> (24.2, 0)
  line L33 (24.2, 0) -> (24.2, 4.05)
  line L34 (24.2, 4.05) -> (20.2, 4.05)
  line L35 (20.2, 4.05) -> (20.2, 7.95)
  line L36 (-0.75, 24) -> (0.75, 24)
  line L37 (0.75, -4) -> (-0.75, -4)
  line L38 (-0.75, 20) -> (-0.75, 19.1)
  line L39 (-0.75, 19.1) -> (-1.5, 19.1)
  line L40 (-1.5, 19.1) -> (-1.5, 17.9)
  line L41 (-1.5, 17.9) -> (1.5, 17.9)
  line L42 (1.5, 17.9) -> (1.5, 19.1)
  line L43 (1.5, 19.1) -> (0.75, 19.1)
  line L44 (0.75, 19.1) -> (0.75, 20)
  line L45 (0.75, 0) -> (0.75, 0.9)
  line L46 (0.75, 0.9) -> (1.5, 0.9)
  line L47 (1.5, 0.9) -> (1.5, 2.1)
  line L48 (1.5, 2.1) -> (-1.5, 2.1)
  line L49 (-1.5, 2.1) -> (-1.5, 0.9)
  line L50 (-1.5, 0.9) -> (-0.75, 0.9)
  line L51 (-0.75, 0.9) -> (-0.75, 0)
  dimension "d288" = 1.2
  dimension "d289" = 3
  dimension "d290" = 6.1
  dimension "d291" = 1.2
  dimension "d292" = 3
  dimension "d293" = 6.1
  constraint coincident L10 L38.start
  constraint perpendicular L10 L38
  constraint perpendicular L38 L39
  constraint perpendicular L39 L40
  constraint perpendicular L40 L41
  constraint perpendicular L41 L42
  constraint perpendicular L42 L43
  constraint perpendicular L10 L44
  constraint coincident L10 L44.end
  constraint coincident L36.end L44
  constraint coincident L36.start L38
  constraint coincident L28 L45.start
  constraint perpendicular L28 L45
  constraint perpendicular L45 L46
  constraint perpendicular L28 L47
  constraint perpendicular L47 L48
  constraint perpendicular L48 L49
  constraint perpendicular L49 L50
  constraint perpendicular L28 L51
  constraint coincident L28 L51.end
  constraint coincident L37.end L51
  constraint coincident L37.start L45
  constraint equal L46 L50
  constraint equal L39 L43
  constraint collinear L39 L43
  constraint collinear L46 L50
  measures "d288" distance of L46.end L47.end
  measures "d289" distance of L47.end L48.end
  measures "d290" distance of L37 L48
  measures "d291" distance of L41.end L42.end
  measures "d292" distance of L40.end L41.end
  measures "d293" distance of L36 L41
extrude "Extrude42" cut sketch "Sketch31" against normal through all contours L28 L45 L46 L47 L48 L49 L50 L51 | L10 L38 L39 L40 L41 L42 L43 L44 bodies 2 4
ref_plane "WorkPlane3" through (0, 10, 0) normal (0, 1, 0) x (0, 0, 1)
sketch "Sketch32" plane through (0, 10, 0) normal (0, 1, 0) x (1, 0, 0)
  line L0 (20.2, 25.2) -> (-20.2, 25.2)
  line L1 (-20.2, 25.2) -> (-20.2, -25.2)
  line L2 (-20.2, -25.2) -> (20.2, -25.2)
  line L3 (20.2, -25.2) -> (20.2, 25.2)
  line L4 (20.2, 25.2) -> (-20.2, -25.2) construction
  line L5 (-20.2, 25.2) -> (20.2, -25.2) construction
  line L6 (8, 25.2) -> (12, 25.2)
  line L7 (12, 25.2) -> (12, 29.2)
  line L8 (12, 29.2) -> (8, 29.2)
  line L9 (8, 29.2) -> (8, 25.2)
  line L10 (0, 25.2) -> (0, 27.8821) construction
  line L11 (-12, -25.2) -> (-8, -25.2)
  line L12 (-8, -25.2) -> (-8, -29.2)
  line L13 (-8, -29.2) -> (-12, -29.2)
  line L14 (-12, -29.2) -> (-12, -25.2)
  line L15 (20.2, -8) -> (24.2, -8)
  line L16 (24.2, -8) -> (24.2, -12)
  line L17 (24.2, -12) -> (20.2, -12)
  line L18 (20.2, -12) -> (20.2, -8)
  line L19 (-24.2, 12) -> (-20.2, 12)
  line L20 (-20.2, 12) -> (-20.2, 8)
  line L21 (-20.2, 8) -> (-24.2, 8)
  line L22 (-24.2, 8) -> (-24.2, 12)
  line L23 (20.2, 0) -> (23.3811, 0) construction
  line L24 (-20.2, 0) -> (-23.5647, 0) construction
  line L25 (0, -25.2) -> (0, -28.4884) construction
  dimension "d306" = 40.4
  dimension "d307" = 50.4
  dimension "d308" = 4
  dimension "d309" = 4
  dimension "d310" = 8
  dimension "d311" = 4
  dimension "d312" = 4
  dimension "d313" = 4
  dimension "d314" = 4
  dimension "d315" = 4
  dimension "d316" = 4
  dimension "d317" = 8
  dimension "d318" = 8
  dimension "d319" = 8
  constraint perpendicular L0 L1
  constraint parallel L0 L2
  constraint parallel L1 L3
  constraint horizontal L0
  constraint coincident L4 origin
  constraint coincident L5 origin
  constraint horizontal L6
  constraint vertical L7
  constraint horizontal L8
  constraint vertical L9
  constraint collinear L0 L6
  constraint midpoint L0 L10.start
  constraint perpendicular L0 L10
  constraint horizontal L11
  constraint vertical L12
  constraint horizontal L13
  constraint vertical L14
  constraint horizontal L15
  constraint vertical L16
  constraint horizontal L17
  constraint vertical L18
  constraint horizontal L19
  constraint vertical L20
  constraint horizontal L21
  constraint vertical L22
  constraint collinear L1 L20
  constraint collinear L2 L11
  constraint collinear L3 L18
  constraint midpoint L3 L23.start
  constraint perpendicular L3 L23
  constraint midpoint L1 L24.start
  constraint perpendicular L1 L24
  constraint midpoint L2 L25.start
  constraint perpendicular L2 L25
  measures "d306" distance of L0.start L0.end
  measures "d307" distance of L0.start L2.end
  measures "d308" distance of L7.end L8.end
  measures "d309" distance of L6.start L8.end
  measures "d310" distance of L9 L10
  measures "d311" distance of L15.start L15.end
  measures "d312" distance of L11.end L12.end
  measures "d313" distance of L20.end L21.end
  measures "d314" distance of L19.start L21.end
  measures "d315" distance of L12.end L13.end
  measures "d316" distance of L15.end L16.end
  measures "d317" distance of L12 L25
  measures "d318" distance of L15 L23
  measures "d319" distance of L21 L24
extrude "Extrude43" add sketch "Sketch32" along normal blind 4 separate body makes body 7
combine "Combine2" operation cut target body 2 tool bodies 7 keep tools
combine "Combine3" operation cut target body 6 tool bodies 7 keep tools
combine "Combine4" operation cut target body 4 tool bodies 7 keep tools
combine "Combine5" operation cut target body 5 tool bodies 7 keep tools
equation "d4 = d9 + d3"
equation "d15 = -d9"
equation "d19 = d225"
equation "d21 = d9"
equation "d74 = d199"
equation "d75 = d74"
equation "d76 = d74"
equation "d77 = d74"
equation "d78 = d74"
equation "d79 = d78"
equation "d80 = d78"
equation "d81 = d78"
equation "d82 = d80"
equation "d83 = d80"
equation "d84 = d82"
equation "d85 = d84"
equation "d86 = d74"
equation "d87 = d86"
equation "d88 = d87"
equation "d91 = d9"
equation "d161 = 68.40 mm / 6"
equation "d198 = d86"
equation "d210 = d199"
equation "d226 = -d9"
equation "d228 = -d9"
equation "d231 = d199"
equation "d232 = d199"
equation "d235 = d9"
equation "d239 = d238"
equation "d240 = d238"
equation "d241 = d240"
equation "d242 = d241"
equation "d243 = d242"
equation "d244 = d243"
equation "d245 = d242"
equation "d246 = d244"
equation "d247 = d246"
equation "d248 = d247"
equation "d249 = d248"
equation "d250 = d249"
equation "d251 = d250"
equation "d252 = d251"
equation "d253 = d252"
equation "d257 = -d225"
equation "d258 = -d9"
equation "d260 = d238"
equation "d261 = d260"
equation "d262 = d261"
equation "d263 = d262"
equation "d266 = d141"
equation "d267 = -d9"
equation "d269 = -d9"
equation "d272 = d275"
equation "d276 = d273"
equation "d277 = d274"
equation "d278 = d272"
equation "d279 = d277"
equation "d280 = d276"
equation "d281 = d280"
equation "d282 = d279"
equation "d283 = d278"
equation "d284 = d278"
equation "d285 = d279"
equation "d286 = d280"
equation "d288 = d274"
equation "d289 = d275"
equation "d290 = d273"
equation "d291 = d288"
equation "d292 = d289"
equation "d293 = d290"
equation "d296 = d231"
equation "d298 = d9"
equation "d299 = d9"
equation "d300 = d9"
equation "d301 = d9"
equation "d303 = d296"
equation "d304 = d231"
equation "d306 = d2 + 2 * d3"
equation "d307 = d1 + 2 * d3"
equation "d308 = d199"
equation "d309 = d9"
equation "d310 = d308 * 2"
equation "d311 = d309"
equation "d312 = d309"
equation "d313 = d309"
equation "d314 = d308"
equation "d315 = d308"
equation "d316 = d308"
equation "d317 = d310"
equation "d318 = d310"
equation "d319 = d310"
equation "d320 = d9"
